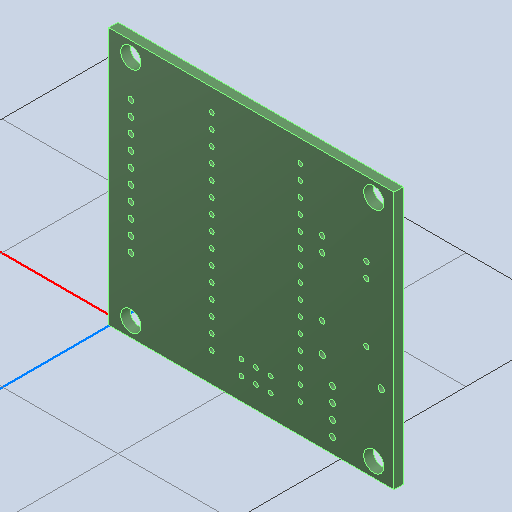
# Autodesk Inventor part: BATTERIES_CONTROLLER.brdКонтур
Saved by Autodesk Inventor 2022 (Build 260153000, 153)
## iProperties
Created: 2022-12-23
Part Number: BATTERIES_CONTROLLER.brdКонтур
Material: Типовые
Document SubType Name: Modeling
Designer: Ivan Petrov
Density: 1 g/cm^3
Appearance: Контур панели
Author: Ivan Petrov
Autodesk Inventor part; units mm, degrees
ref_plane "YZ Plane" through (0, 0, 0) normal (1, 0, 0) x (0, 1, 0)
ref_plane "XZ Plane" through (0, 0, 0) normal (0, 1, 0) x (-1, 0, 0)
ref_plane "XY Plane" through (0, 0, 0) normal (0, 0, 1) x (1, 0, 0)
sketch "Эскиз1" plane through (0, 0, 0) normal (0, 0, 1) x (1, 0, 0)
  line L0 (0, 0) -> (49.2, 0)
  line L1 (49.2, 0) -> (49.2, 44.44)
  line L2 (49.2, 44.44) -> (0, 44.44)
  line L3 (0, 44.44) -> (0, 0)
  circle A0 centre (36.83, 13.97) radius 0.56
  circle A1 centre (46.99, 13.97) radius 0.56
  circle A2 centre (3.81, 12.7) radius 0.5
  circle A3 centre (3.81, 15.24) radius 0.5
  circle A4 centre (3.81, 17.78) radius 0.5
  circle A5 centre (3.81, 20.32) radius 0.5
  circle A6 centre (3.81, 22.86) radius 0.5
  circle A7 centre (3.81, 25.4) radius 0.5
  circle A8 centre (3.81, 27.94) radius 0.5
  circle A9 centre (3.81, 30.48) radius 0.5
  circle A10 centre (3.81, 33.02) radius 0.5
  circle A11 centre (3.81, 35.56) radius 0.5
  circle A12 centre (38.58, 10.2) radius 0.51
  circle A13 centre (38.58, 7.66) radius 0.51
  circle A14 centre (38.58, 5.12) radius 0.51
  circle A15 centre (38.58, 2.58) radius 0.51
  circle A16 centre (44.45, 29.21) radius 0.455
  circle A17 centre (36.83, 29.21) radius 0.455
  circle A18 centre (36.83, 31.75) radius 0.455
  circle A19 centre (44.45, 19.05) radius 0.455
  circle A20 centre (36.83, 19.05) radius 0.455
  circle A21 centre (44.45, 31.75) radius 0.455
  circle A22 centre (17.78, 38.1) radius 0.4
  circle A23 centre (17.78, 12.7) radius 0.4
  circle A24 centre (17.78, 33.02) radius 0.4
  circle A25 centre (17.78, 30.48) radius 0.4
  circle A26 centre (17.78, 27.94) radius 0.4
  circle A27 centre (17.78, 25.4) radius 0.4
  circle A28 centre (17.78, 22.86) radius 0.4
  circle A29 centre (17.78, 20.32) radius 0.4
  circle A30 centre (17.78, 17.78) radius 0.4
  circle A31 centre (17.78, 15.24) radius 0.4
  circle A32 centre (17.78, 35.56) radius 0.4
  circle A33 centre (33.02, 15.24) radius 0.4
  circle A34 centre (33.02, 17.78) radius 0.4
  circle A35 centre (33.02, 20.32) radius 0.4
  circle A36 centre (33.02, 22.86) radius 0.4
  circle A37 centre (33.02, 25.4) radius 0.4
  circle A38 centre (33.02, 27.94) radius 0.4
  circle A39 centre (33.02, 30.48) radius 0.4
  circle A40 centre (33.02, 33.02) radius 0.4
  circle A41 centre (33.02, 35.56) radius 0.4
  circle A42 centre (33.02, 38.1) radius 0.4
  circle A43 centre (33.02, 40.64) radius 0.4
  circle A44 centre (17.78, 40.64) radius 0.4
  circle A45 centre (17.78, 7.62) radius 0.4
  circle A46 centre (33.02, 12.7) radius 0.4
  circle A47 centre (22.86, 3.81) radius 0.4
  circle A48 centre (22.86, 6.35) radius 0.4
  circle A49 centre (25.4, 3.81) radius 0.4
  circle A50 centre (25.4, 6.35) radius 0.4
  circle A51 centre (27.94, 3.81) radius 0.4
  circle A52 centre (27.94, 6.35) radius 0.4
  circle A53 centre (17.78, 5.08) radius 0.4
  circle A54 centre (17.78, 10.16) radius 0.4
  circle A55 centre (33.02, 10.16) radius 0.4
  circle A56 centre (33.02, 7.62) radius 0.4
  circle A57 centre (33.02, 5.08) radius 0.4
  circle A58 centre (3.81, 41.91) radius 1.75
  circle A59 centre (3.81, 2.54) radius 1.75
  circle A60 centre (45.72, 2.54) radius 1.75
  circle A61 centre (45.72, 41.91) radius 1.75
  constraints: 62 centre point, 8 end point
extrude "BATTERIES_CONTROLLER.brdКонтур" add sketch "Эскиз1" along normal blind 1.6
